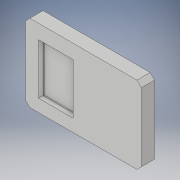
# Autodesk Inventor part: RFID scanner
Saved by Autodesk Inventor 2019 (Build 230136000, 136)
## iProperties
Created: 2020-03-04
Part Number: RFID scanner
Material: Generic
Document SubType Name: Modeling
Designer: hp
Density: 1 g/cm^3
Appearance: Default
Author: hp
Autodesk Inventor part; units mm, degrees
ref_plane "YZ Plane" through (0, 0, 0) normal (1, 0, 0) x (0, 1, 0)
ref_plane "XZ Plane" through (0, 0, 0) normal (0, 1, 0) x (-1, 0, 0)
ref_plane "XY Plane" through (0, 0, 0) normal (0, 0, 1) x (1, 0, 0)
sketch "Sketch1" plane through (0, 0, 0) normal (0, 0, 1) x (1, 0, 0)
  line L0 (-12.2838, 5.95) -> (-117.2838, 5.95)
  line L1 (-117.2838, 5.95) -> (-117.2838, -64.05)
  line L2 (-117.2838, -64.05) -> (-12.2838, -64.05)
  line L3 (-12.2838, -64.05) -> (-12.2838, 5.95)
  point P0 (0, 0)
  dimension "d0" = 105
  dimension "d1" = 70
  constraints: 8 end point, 2 parallel, 1 horizontal, 1 perpendicular
  measures "d0" distance of L2.end L1.end
  measures "d1" distance of L1.end L0.end
extrude "Extrusion1" add sketch "Sketch1" along normal blind 12
chamfer "Chamfer1" distance 4 angle 45 4 edges at (-12.2838, 5.95, 6) (-12.2838, -64.05, 6) (-117.2838, -64.05, 6) (-117.2838, 5.95, 6)
sketch "Sketch2" plane through (0, 0, 12) normal (0, 0, 1) x (1, 0, 0)
  line L0 (-103.2855, -8.853) -> (-76.1362, -8.853)
  line L1 (-76.1362, -8.853) -> (-76.1362, -50.7574)
  line L2 (-76.1362, -50.7574) -> (-103.2855, -50.7574)
  line L3 (-103.2855, -50.7574) -> (-103.2855, -8.853)
  point P0 (0, 0)
  constraints: 8 end point, 2 parallel, 1 horizontal, 1 perpendicular
extrude "Extrusion2" cut sketch "Sketch2" against normal blind 3
chamfer "Chamfer2" distance 2 angle 45 4 edges at (-103.2855, -29.8052, 12) (-89.7108, -8.853, 12) (-76.1362, -29.8052, 12) (-89.7108, -50.7574, 12)
body "Solid1"
